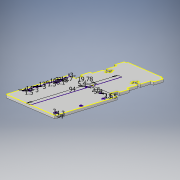
# Autodesk Inventor part: 板子9
Saved by Autodesk Inventor 2017 (Build 210142000, 142)
## iProperties
Part Number: 板子9
Material: 一般
Document SubType Name: Modeling
Designer: User
Density: 1 g/cm^3
Appearance: 預設
Author: User
Autodesk Inventor part; units mm, degrees
ref_plane "YZ Plane" through (0, 0, 0) normal (1, 0, 0) x (0, 1, 0)
ref_plane "XZ Plane" through (0, 0, 0) normal (0, 1, 0) x (-1, 0, 0)
ref_plane "XY Plane" through (0, 0, 0) normal (0, 0, 1) x (1, 0, 0)
sketch "草圖1" plane through (0, 0, 0) normal (0, 1, 0) x (-1, 0, 0)
  line L0 (42, 0) -> (-42, 0) projected
  line L1 (0, -77.6) -> (0, 87.6) projected
  line L2 (-30, 0) -> (-30, 64)
  line L3 (-30, 64) -> (30, 64)
  line L4 (30, 64) -> (30, 0)
  line L5 (21, 0) -> (21, -7.5)
  line L6 (21, -7.5) -> (0, -7.5)
  line L7 (0, -7.5) -> (24, -7.5)
  line L8 (24, -7.5) -> (24, -17.5)
  line L9 (24, -17.5) -> (0, -17.5)
  line L10 (0, -17.5) -> (0, -7.5)
  line L11 (0, -17.5) -> (21, -17.5)
  line L12 (21, -17.5) -> (21, -42.5)
  line L13 (21, -42.5) -> (0, -42.5)
  line L14 (0, -42.5) -> (0, -17.5)
  line L15 (0, -42.5) -> (24, -42.5)
  line L16 (24, -42.5) -> (24, -52.5)
  line L17 (24, -52.5) -> (0, -52.5)
  line L18 (0, -52.5) -> (0, -42.5)
  line L19 (0, -52.5) -> (21, -52.5)
  line L20 (21, -52.5) -> (21, -54)
  line L21 (21, -54) -> (0, -54)
  line L22 (0, -54) -> (0, -52.5)
  line L23 (-21, 0) -> (-21, -7.5)
  line L24 (-21, -7.5) -> (0, -7.5)
  line L25 (0, -7.5) -> (-24, -7.5)
  line L26 (-24, -7.5) -> (-24, -17.5)
  line L27 (-24, -17.5) -> (0, -17.5)
  line L28 (0, -17.5) -> (-21, -17.5)
  line L29 (-21, -17.5) -> (-21, -42.5)
  line L30 (-21, -42.5) -> (0, -42.5)
  line L31 (0, -42.5) -> (-24, -42.5)
  line L32 (-24, -42.5) -> (-24, -52.5)
  line L33 (-24, -52.5) -> (0, -52.5)
  line L34 (0, -52.5) -> (-21, -52.5)
  line L35 (-21, -52.5) -> (-21, -54)
  line L36 (-21, -54) -> (0, -54)
  line L37 (30, 0) -> (21, 0)
  line L38 (-21, 0) -> (-30, 0)
  point P0 (0, 0)
  dimension "d0" = 60
  dimension "d1" = 64
  dimension "d2" = 30
  dimension "d3" = 9
  dimension "d4" = 7.5
  dimension "d5" = 10
  dimension "d6" = 3
  dimension "d7" = 25
  dimension "d8" = 10
  dimension "d9" = 3
  dimension "d10" = 9
  dimension "d11" = 1.5
  constraints: 74 end point, 11 parallel, 10 symmetric about line, 6 horizontal, 6 perpendicular, 3 point on line
  measures "d0" distance of L2.end L3.end
  measures "d1" distance of L2.start L2.end
  measures "d2" distance between parallel lines of L1 L4
  measures "d3" distance between parallel lines of L5 L4
  measures "d4" distance of L5.start L5.end
  measures "d5" distance of L7.end L8.end
  measures "d6" distance between parallel lines of L12 L8
  measures "d7" distance of L11.end L12.end
  measures "d8" distance of L15.end L16.end
  measures "d9" distance between parallel lines of L12 L16
  measures "d10" distance between parallel lines of L4 L20
  measures "d11" distance of L19.end L20.end
extrude "擠出1" add sketch "草圖1" along normal mid plane 3
sketch "草圖2" plane through (0, 1.5, 0) normal (0, 1, 0) x (1, 0, 0)
  line L0 (-21, 52.5) -> (-21, 54) projected
  line L1 (-21, 54) -> (21, 54) projected
  line L2 (21, 54) -> (21, 52.5) projected
  line L3 (21, 52.5) -> (24, 52.5) projected
  line L4 (24, 52.5) -> (24, 42.5) projected
  line L5 (24, 42.5) -> (21, 42.5) projected
  line L6 (21, 42.5) -> (21, 17.5) projected
  line L7 (21, 17.5) -> (24, 17.5) projected
  line L8 (24, 17.5) -> (24, 7.5) projected
  line L9 (24, 7.5) -> (21, 7.5) projected
  line L10 (21, 7.5) -> (21, 0) projected
  line L11 (21, 0) -> (30, 0) projected
  line L12 (30, 0) -> (30, -64) projected
  line L13 (30, -64) -> (-30, -64) projected
  line L14 (-30, -64) -> (-30, 0) projected
  line L15 (-30, 0) -> (-21, 0) projected
  line L16 (-21, 0) -> (-21, 7.5) projected
  line L17 (-21, 7.5) -> (-24, 7.5) projected
  line L18 (-24, 7.5) -> (-24, 17.5) projected
  line L19 (-24, 17.5) -> (-21, 17.5) projected
  line L20 (-21, 17.5) -> (-21, 42.5) projected
  line L21 (-21, 42.5) -> (-24, 42.5) projected
  line L22 (-24, 42.5) -> (-24, 52.5) projected
  line L23 (-24, 52.5) -> (-21, 52.5) projected
  line L24 (-21, 28.5) -> (-17, 28.5)
  line L25 (-17, 28.5) -> (-17, 31.5)
  line L26 (-17, 31.5) -> (-21, 31.5)
  line L27 (-21, 31.5) -> (-21, 28.5)
  line L28 (-17, 26) -> (-14.5, 26)
  line L29 (-14.5, 26) -> (-14.5, 34)
  line L30 (-14.5, 34) -> (-17, 34)
  line L31 (-17, 34) -> (-17, 26)
  line L32 (-14.5, 28.5) -> (-13, 28.5)
  line L33 (-13, 28.5) -> (-13, 31.5)
  line L34 (-13, 31.5) -> (-14.5, 31.5)
  line L35 (-14.5, 31.5) -> (-14.5, 28.5)
  line L36 (0, 0) -> (0, 17.5)
  line L37 (21, 28.5) -> (17, 28.5)
  line L38 (17, 28.5) -> (17, 31.5)
  line L39 (17, 31.5) -> (21, 31.5)
  line L40 (17, 26) -> (14.5, 26)
  line L41 (14.5, 26) -> (14.5, 34)
  line L42 (14.5, 34) -> (17, 34)
  line L43 (17, 34) -> (17, 26)
  line L44 (14.5, 28.5) -> (13, 28.5)
  line L45 (13, 28.5) -> (13, 31.5)
  line L46 (13, 31.5) -> (14.5, 31.5)
  line L47 (14.5, 31.5) -> (14.5, 28.5)
  line L48 (21, 28.5) -> (21, 31.5)
  line L49 (21, 42.5) -> (21, 17.5) projected
  dimension "d14" = 3
  dimension "d15" = 11
  dimension "d16" = 4
  dimension "d17" = 2.5
  dimension "d18" = 1.5
  dimension "d19" = 2.5
  dimension "d20" = 2.5
  constraints: 50 end point, 12 symmetric about line, 9 point on line, 6 parallel, 3 horizontal, 3 perpendicular, 1 collinear, 1 vertical
  measures "d14" distance between parallel lines of L26 L24
  measures "d15" distance between parallel lines of L19 L24
  measures "d16" distance of L24.start L24.end
  measures "d17" distance of L28.start L28.end
  measures "d18" distance of L32.start L32.end
  measures "d19" distance between parallel lines of L24 L28
  measures "d20" distance between parallel lines of L34 L30
extrude "擠出2" cut sketch "草圖2" against normal blind 10 contours L26 L25 L24 L20 | L31 L30 L29 L28 L25 | L6 L37 L38 L39 | L38 L43 L40 L41 L42 | L34 L33 L32 L29 | L41 L44 L45 L46
sketch "草圖3" plane through (0, 1.5, 0) normal (0, 1, 0) x (1, 0, 0)
  line L0 (-21, 28.5) -> (-17, 28.5) projected
  line L1 (-17, 28.5) -> (-17, 26) projected
  line L2 (-17, 26) -> (-14.5, 26) projected
  line L3 (-14.5, 26) -> (-14.5, 28.5) projected
  line L4 (-14.5, 28.5) -> (-13, 28.5) projected
  line L5 (-13, 28.5) -> (-13, 31.5) projected
  line L6 (-13, 31.5) -> (-14.5, 31.5) projected
  line L7 (-14.5, 31.5) -> (-14.5, 34) projected
  line L8 (-14.5, 34) -> (-17, 34) projected
  line L9 (-17, 34) -> (-17, 31.5) projected
  line L10 (-17, 31.5) -> (-21, 31.5) projected
  line L11 (-21, 31.5) -> (-21, 42.5) projected
  line L12 (-21, 42.5) -> (-24, 42.5) projected
  line L13 (-24, 42.5) -> (-24, 52.5) projected
  line L14 (-24, 52.5) -> (-21, 52.5) projected
  line L15 (-21, 52.5) -> (-21, 54) projected
  line L16 (-21, 54) -> (21, 54) projected
  line L17 (21, 54) -> (21, 52.5) projected
  line L18 (21, 52.5) -> (24, 52.5) projected
  line L19 (24, 52.5) -> (24, 42.5) projected
  line L20 (24, 42.5) -> (21, 42.5) projected
  line L21 (21, 42.5) -> (21, 31.5) projected
  line L22 (21, 31.5) -> (17, 31.5) projected
  line L23 (17, 31.5) -> (17, 34) projected
  line L24 (17, 34) -> (14.5, 34) projected
  line L25 (14.5, 34) -> (14.5, 31.5) projected
  line L26 (14.5, 31.5) -> (13, 31.5) projected
  line L27 (13, 31.5) -> (13, 28.5) projected
  line L28 (13, 28.5) -> (14.5, 28.5) projected
  line L29 (14.5, 28.5) -> (14.5, 26) projected
  line L30 (14.5, 26) -> (17, 26) projected
  line L31 (17, 26) -> (17, 28.5) projected
  line L32 (17, 28.5) -> (21, 28.5) projected
  line L33 (21, 28.5) -> (21, 17.5) projected
  line L34 (21, 17.5) -> (24, 17.5) projected
  line L35 (24, 17.5) -> (24, 7.5) projected
  line L36 (24, 7.5) -> (21, 7.5) projected
  line L37 (21, 7.5) -> (21, 0) projected
  line L38 (21, 0) -> (30, 0) projected
  line L39 (30, 0) -> (30, -64) projected
  line L40 (30, -64) -> (-30, -64) projected
  line L41 (-30, -64) -> (-30, 0) projected
  line L42 (-30, 0) -> (-21, 0) projected
  line L43 (-21, 0) -> (-21, 7.5) projected
  line L44 (-21, 7.5) -> (-24, 7.5) projected
  line L45 (-24, 7.5) -> (-24, 17.5) projected
  line L46 (-24, 17.5) -> (-21, 17.5) projected
  line L47 (-21, 17.5) -> (-21, 28.5) projected
  line L48 (-30, 0) -> (-21, 0) projected
  line L49 (-30, 0) -> (-27, 0)
  line L50 (-27, 0) -> (-27, -11.7)
  line L51 (-27, -11.7) -> (-24.2, -11.7)
  line L52 (-24.2, -11.7) -> (-24.2, -16.8)
  circle A0 centre (-27, -11.7) radius 1.5
  circle A1 centre (-24.2, -16.8) radius 1.5
  line L53 (-27, -11.7) -> (-27, -21.7)
  circle A2 centre (-27, -21.7) radius 0.75
  line L54 (-27, -21.7) -> (-27, -34.7)
  circle A3 centre (-27, -34.7) radius 1.5
  line L55 (-27, -34.7) -> (-27, -48.7)
  circle A4 centre (-27, -48.7) radius 0.75
  line L56 (-27, -48.7) -> (-27, -44.7)
  line L57 (-27, -44.7) -> (-24.2, -44.7)
  circle A5 centre (-24.2, -44.7) radius 1.5
  line L58 (30, -64) -> (-30, -64) projected
  line L59 (0, -64) -> (0, 30)
  circle A6 centre (27, -11.7) radius 1.5
  circle A7 centre (27, -34.7) radius 1.5
  circle A8 centre (25.7, -60) radius 1.5
  circle A9 centre (16.5, -5.4) radius 1.3
  circle A10 centre (-1.22, -5.4) radius 1.3
  point P0 (0, 0)
  dimension "d23" = 3
  dimension "d24" = 11.7
  dimension "d25" = 2.8
  dimension "d26" = 5.1
  dimension "d27" = 3
  dimension "d28" = 3
  dimension "d29" = 10
  dimension "d30" = 1.5
  dimension "d31" = 13
  dimension "d32" = 3
  dimension "d33" = 14
  dimension "d34" = 1.5
  dimension "d35" = 4
  dimension "d36" = 3
  dimension "d37" = 94
  dimension "d38" = 4.3
  dimension "d39" = 4
  dimension "d40" = 3
  dimension "d41" = 2.6
  dimension "d42" = 5.4
  dimension "d43" = 13.5
  dimension "d44" = 2.6
  dimension "d45" = 19.78
  dimension "d46" = 5.4
  constraints: 20 end point, 11 centre point, 6 coincident, 4 vertical, 3 perpendicular, 3 point on line, 2 symmetric about line, 1 horizontal, 1 midpoint, 2 other
  measures "d23" distance of L41.end L49.end
  measures "d24" distance of L49.end L50.end
  measures "d25" distance of L50.end L51.end
  measures "d26" distance of L51.end L52.end
  measures "d27" diameter of A0
  measures "d28" diameter of A1
  measures "d29" distance of L53.start L53.end
  measures "d30" diameter of A2
  measures "d31" distance of L54.start L54.end
  measures "d32" diameter of A3
  measures "d33" distance of L55.start L55.end
  measures "d34" diameter of A4
  measures "d35" distance of L56.start L56.end
  measures "d36" diameter of A5
  measures "d37" distance of L59.start L59.end
  measures "d38" distance from line of L39 A8.centre
  measures "d39" distance from line of L40 A8.centre
  measures "d40" diameter of A8
  measures "d41" diameter of A9
  measures "d42" vertical distance of L37.end A9.centre
  measures "d43" distance from line of L39 A9.centre
  measures "d44" diameter of A10
  measures "d45" horizontal distance of L42.end A10.centre
  measures "d46" vertical distance of L37.end A10.centre
